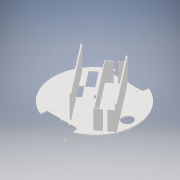
# Autodesk Inventor part: DonjaKonstrukcija_v.5.0
Saved by Autodesk Inventor 2020 (Build 240168000, 168)
## iProperties
Created: 2020-12-12
Part Number: DonjaKonstrukcija_v.5.0
Material: Generic
Document SubType Name: Modeling
Designer: Sičaja
Density: 1 g/cm^3
Appearance: Default
Author: Sičaja
Autodesk Inventor part; units mm, degrees
ref_plane "YZ Plane" through (0, 0, 0) normal (1, 0, 0) x (0, 1, 0)
ref_plane "XZ Plane" through (0, 0, 0) normal (0, 1, 0) x (-1, 0, 0)
ref_plane "XY Plane" through (0, 0, 0) normal (0, 0, 1) x (1, 0, 0)
sketch "Sketch1" plane through (0, 0, 0) normal (0, 1, 0) x (-1, 0, 0)
  arc A0 (125.0036, -29.4917) -> (126.5876, -26.2706) centre (125.0036, -27.4917) ccw projected
  line L0 (126.5876, -26.2706) -> (124.622, -23.7208) projected
  arc A1 (124.622, -23.7208) -> (122.2517, -23.1029) centre (123.038, -24.9419) ccw projected
  arc A2 (119.8815, -22.485) -> (122.2517, -23.1029) centre (121.4655, -21.264) ccw projected
  line L1 (119.8815, -22.485) -> (109.257, -8.7027) projected
  arc A3 (109.257, -8.7027) -> (107.673, -7.9237) centre (107.673, -9.9237) ccw projected
  line L2 (107.673, -7.9237) -> (105.1478, -7.9237) projected
  arc A4 (105.1478, -7.9237) -> (103.5638, -11.1448) centre (105.1478, -9.9237) ccw projected
  line L3 (103.5638, -11.1448) -> (117.1065, -28.7128) projected
  arc A5 (117.1065, -28.7128) -> (118.6904, -29.4917) centre (118.6904, -27.4917) ccw projected
  line L4 (118.6904, -29.4917) -> (125.0036, -29.4917) projected
  arc A6 (88.5004, 50.076) -> (88.5004, -87.4914) centre (118.3968, -18.7077) ccw projected
  line L5 (88.5004, 50.076) -> (90.9141, 40.0763) projected
  line L6 (90.9141, 40.0763) -> (103.8135, 40.0763) projected
  line L7 (103.8135, 40.0763) -> (103.8135, 42.0763) projected
  line L8 (103.8135, 42.0763) -> (105.8135, 42.0763) projected
  line L9 (105.8135, 42.0763) -> (105.8135, 40.0763) projected
  line L10 (105.8135, 40.0763) -> (117.3968, 40.0763) projected
  line L11 (117.3968, 40.0763) -> (117.3968, 42.0763) projected
  line L12 (117.3968, 42.0763) -> (119.3968, 42.0763) projected
  line L13 (119.3968, 42.0763) -> (119.3968, 40.0763) projected
  line L14 (119.3968, 40.0763) -> (145.8796, 40.0763) projected
  line L15 (145.8796, 40.0763) -> (148.2933, 50.076) projected
  arc A7 (148.2933, -87.4914) -> (148.2933, 50.076) centre (118.3968, -18.7077) ccw projected
  line L16 (148.2933, -87.4914) -> (145.8796, -77.4917) projected
  line L17 (145.8796, -77.4917) -> (119.3968, -77.4917) projected
  line L18 (119.3968, -77.4917) -> (119.3968, -79.4917) projected
  line L19 (119.3968, -79.4917) -> (117.3968, -79.4917) projected
  line L20 (117.3968, -79.4917) -> (117.3968, -77.4917) projected
  line L21 (117.3968, -77.4917) -> (90.9141, -77.4917) projected
  line L22 (90.9141, -77.4917) -> (88.5004, -87.4914) projected
  arc A8 (159.9383, -25.3226) -> (160.3012, -22.5175) centre (158.7173, -23.7386) ccw projected
  line L23 (160.3012, -22.5175) -> (147.6614, -6.1208) projected
  arc A9 (147.6614, -6.1208) -> (144.8563, -5.7578) centre (146.0774, -7.3418) ccw projected
  line L24 (144.8563, -5.7578) -> (136.9424, -11.8585) projected
  arc A10 (136.9424, -11.8585) -> (136.5795, -14.6635) centre (138.1635, -13.4424) ccw projected
  line L25 (136.5795, -14.6635) -> (149.2193, -31.0603) projected
  arc A11 (149.2193, -31.0603) -> (152.0244, -31.4232) centre (150.8033, -29.8392) ccw projected
  line L26 (152.0244, -31.4232) -> (159.9383, -25.3226) projected
  line L27 (160.2581, -68.311) -> (170.554, -60.3742) projected
  line L28 (170.554, -60.3742) -> (149.198, -32.6705) projected
  line L29 (149.198, -32.6705) -> (138.9021, -40.6074) projected
  line L30 (138.9021, -40.6074) -> (160.2581, -68.311) projected
  circle A12 centre (95.126, 34.6643) radius 1 projected
  circle A13 centre (141.6676, -72.0797) radius 1 projected
  circle A14 centre (141.6676, 34.6643) radius 1 projected
  circle A15 centre (95.126, -72.0797) radius 1 projected
  line L31 (108.9507, 33.0198) -> (177.0722, -55.3494) projected
  line L32 (177.0722, -55.3494) -> (178.6562, -54.1284) projected
  line L33 (178.6562, -54.1284) -> (110.5346, 34.2409) projected
  line L34 (110.5346, 34.2409) -> (108.9507, 33.0198) projected
  point P0 (0, 0)
extrude "DnoKonstrukcije" add sketch "Sketch1" along normal blind 2 contours L5 L6 L7 L8 L9 L10 L11 L12 L13 L14 L15 A7 L16 L17 L18 L19 L20 L21 L22 A6 | L33 L32 L31 L26 | L24 L31 L34 L33
sketch "Sketch6" plane through (0, 2, 0) normal (0, 1, 0) x (1, 0, 0)
  line L0 (-63.4991, -21.1731) -> (-64.1097, -20.3811) projected
  line L1 (-64.1097, -20.3811) -> (-72.8216, -27.0969) projected
  line L2 (-72.8216, -27.0969) -> (-137.5376, 56.8545) projected
  line L3 (-137.5376, 56.8545) -> (-128.6995, 63.6676) projected
  line L4 (-128.6995, 63.6676) -> (-129.31, 64.4595) projected
  line L5 (-129.31, 64.4595) -> (-138.9401, 57.036) projected
  line L6 (-73.0031, -28.4994) -> (-138.9401, 57.036) projected
  line L7 (-63.4991, -21.1731) -> (-73.0031, -28.4994) projected
  line L8 (-50.8272, -11.4047) -> (-51.4378, -10.6127) projected
  line L9 (-51.4378, -10.6127) -> (-59.3577, -16.7179) projected
  line L10 (-59.3577, -16.7179) -> (-58.7472, -17.5099) projected
  line L11 (-50.8272, -11.4047) -> (-58.7472, -17.5099) projected
  line L12 (-115.1802, 75.3518) -> (-116.7642, 74.1308) projected
  line L13 (-116.7642, 74.1308) -> (-50.8272, -11.4047) projected
  line L14 (-50.8272, -11.4047) -> (-49.2432, -10.1836) projected
  line L15 (-49.2432, -10.1836) -> (-115.1802, 75.3518) projected
  line L16 (-116.1537, 73.3388) -> (-116.7642, 74.1308) projected
  line L17 (-116.7642, 74.1308) -> (-124.6842, 68.0255) projected
  line L18 (-124.6842, 68.0255) -> (-124.0737, 67.2335) projected
  line L19 (-124.0737, 67.2335) -> (-116.1537, 73.3388) projected
  point P0 (0, 0)
extrude "DrzacZaBateriju" add sketch "Sketch6" along normal blind 34
sketch "Sketch7" plane through (0, 36, 0) normal (0, 1, 0) x (1, 0, 0)
  line L0 (-49.2432, -10.1836) -> (-115.1802, 75.3518) projected
  line L1 (-115.1802, 75.3518) -> (-124.6842, 68.0255) projected
  line L2 (-124.6842, 68.0255) -> (-124.0737, 67.2335) projected
  line L3 (-124.0737, 67.2335) -> (-116.1537, 73.3388) projected
  line L4 (-116.1537, 73.3388) -> (-51.4378, -10.6127) projected
  line L5 (-51.4378, -10.6127) -> (-59.3577, -16.7179) projected
  line L6 (-59.3577, -16.7179) -> (-58.7472, -17.5099) projected
  line L7 (-58.7472, -17.5099) -> (-49.2432, -10.1836) projected
  line L8 (-124.0737, 67.2335) -> (-116.1537, 73.3388) projected
  line L9 (-116.1537, 73.3388) -> (-116.7642, 74.1308)
  line L10 (-51.4378, -10.6127) -> (-59.3577, -16.7179) projected
  line L11 (-51.4378, -10.6127) -> (-50.8272, -11.4047)
  line L12 (-58.7472, -17.5099) -> (-49.2432, -10.1836) projected
  point P0 (0, 0)
  constraints: 4 end point, 3 point on line, 1 perpendicular
extrude "DrzacZaTeensy" add sketch "Sketch7" along normal blind 10 contours L7 L11 L4 L9 L1 L0
sketch "Sketch8" plane through (0, 2, 0) normal (0, 1, 0) x (1, 0, 0)
  line L0 (-108.9507, -33.0198) -> (-177.0722, 55.3494) projected
  line L1 (-177.0722, 55.3494) -> (-178.6562, 54.1284) projected
  line L2 (-178.6562, 54.1284) -> (-110.5346, -34.2409) projected
  line L3 (-110.5346, -34.2409) -> (-108.9507, -33.0198) projected
  point P0 (0, 0)
extrude "DrzacZaPDB" add sketch "Sketch8" along normal blind 42
sketch "Sketch10" plane through (-110.5346, 2, 34.2409) normal (-0.7919947, 0, 0.6105279) x (0.6105279, 0, 0.7919947)
  point P0 (40.3659, -2)
sketch "Sketch11" plane through (-110.5346, 2, 34.2409) normal (-0.7919947, 0, 0.6105279) x (0.6105279, 0, 0.7919947)
  circle A0 centre (-42.3, 37.7) radius 1 projected
  circle A1 centre (-2.3, 37.7) radius 1 projected
  circle A2 centre (-42.3, 7.7) radius 1 projected
  point P0 (40.3659, -2)
extrude "RupeZaPDBSEkranom" cut sketch "Sketch11" against normal blind 2
sketch "Sketch12" plane through (-110.5346, 2, 34.2409) normal (-0.7919947, 0, 0.6105279) x (0.6105279, 0, 0.7919947)
  line L0 (-45.4471, 40.0341) -> (-75.4471, 40.0341)
  line L1 (-75.4471, 40.0341) -> (-75.4471, 5.0341)
  line L2 (-75.4471, 5.0341) -> (-45.4471, 5.0341)
  line L3 (-45.4471, 5.0341) -> (-45.4471, 40.0341)
  line L4 (-71.9471, 37.5341) -> (-48.9471, 37.5341)
  line L5 (-47.9471, 36.5341) -> (-47.9471, 8.5341)
  line L6 (-48.9471, 7.5341) -> (-71.9471, 7.5341)
  line L7 (-72.9471, 8.5341) -> (-72.9471, 36.5341)
  circle A0 centre (-72.9471, 37.5341) radius 1
  circle A1 centre (-47.9471, 37.5341) radius 1
  circle A2 centre (-72.9471, 7.5341) radius 1
  circle A3 centre (-47.9471, 7.5341) radius 1
  point P0 (40.3659, -2)
  dimension "d16" = 30
  dimension "d17" = 35
  dimension "d18" = 2.5
  dimension "d19" = 2
  dimension "d20" = 2
  dimension "d21" = 2
  dimension "d22" = 2
  constraints: 16 end point, 8 point on circle, 4 centre point, 4 parallel, 2 perpendicular, 1 horizontal
  measures "d16" distance of L2.end L1.end
  measures "d17" distance of L1.end L0.end
  measures "d18" distance between parallel lines of L0 L4
  measures "d19" diameter of A0
  measures "d20" diameter of A1
  measures "d21" diameter of A2
  measures "d22" diameter of A3
extrude "RupeZaDriverMotora" cut sketch "Sketch12" against normal blind 2 contours A0 | A1 | A2 | A3
sketch "Sketch15" plane through (-110.5346, 2, 34.2409) normal (-0.7919947, 0, 0.6105279) x (0.6105279, 0, 0.7919947)
  line L0 (-110.3095, 40.1713) -> (-80.3095, 40.1713)
  line L1 (-80.3095, 40.1713) -> (-80.3095, 5.1713)
  line L2 (-80.3095, 5.1713) -> (-110.3095, 5.1713)
  line L3 (-110.3095, 5.1713) -> (-110.3095, 40.1713)
  line L4 (-83.8095, 37.6713) -> (-106.8095, 37.6713)
  line L5 (-107.8095, 36.6713) -> (-107.8095, 8.6713)
  line L6 (-106.8095, 7.6713) -> (-83.8095, 7.6713)
  line L7 (-82.8095, 8.6713) -> (-82.8095, 36.6713)
  circle A0 centre (-107.8095, 37.6713) radius 1
  circle A1 centre (-82.8095, 37.6713) radius 1
  circle A2 centre (-107.8095, 7.6713) radius 1
  circle A3 centre (-82.8095, 7.6713) radius 1
  point P0 (40.3659, -2)
  dimension "d25" = 30
  dimension "d26" = 35
  dimension "d27" = 2.5
  dimension "d28" = 2
  dimension "d29" = 2
  dimension "d30" = 2
  dimension "d31" = 2
  constraints: 16 end point, 8 point on circle, 4 centre point, 4 parallel, 2 perpendicular, 1 horizontal
  measures "d25" distance of L1.end L2.end
  measures "d26" distance of L0.end L1.end
  measures "d27" distance between parallel lines of L0 L4
  measures "d28" diameter of A0
  measures "d29" diameter of A1
  measures "d30" diameter of A2
  measures "d31" diameter of A3
extrude "RupeZaPDB" cut sketch "Sketch15" against normal blind 2 contours A1 | A0 | A3 | A2
sketch "Sketch16" plane through (-115.1802, 2, -75.3518) normal (0.7919947, 0, -0.6105279) x (-0.6105279, 0, -0.7919947)
  line L0 (-89.0986, 42.7042) -> (-24.0986, 42.7042)
  line L1 (-24.0986, 42.7042) -> (-24.0986, 7.7042)
  line L2 (-24.0986, 7.7042) -> (-89.0986, 7.7042)
  line L3 (-89.0986, 7.7042) -> (-89.0986, 42.7042)
  line L4 (-85.5986, 10.2042) -> (-27.5986, 10.2042)
  line L5 (-26.5986, 11.2042) -> (-26.5986, 39.2042)
  line L6 (-27.5986, 40.2042) -> (-85.5986, 40.2042)
  line L7 (-86.5986, 39.2042) -> (-86.5986, 11.2042)
  circle A0 centre (-86.5986, 40.2042) radius 1
  circle A1 centre (-26.5986, 40.2042) radius 1
  circle A2 centre (-86.5986, 10.2042) radius 1
  circle A3 centre (-26.5986, 10.2042) radius 1
  point P0 (-129.999, -2)
  dimension "d34" = 65
  dimension "d35" = 35
  dimension "d36" = 2.5
  dimension "d37" = 2
  dimension "d38" = 2
  dimension "d39" = 2
  dimension "d40" = 2
  constraints: 16 end point, 8 point on circle, 4 centre point, 4 parallel, 2 perpendicular, 1 horizontal
  measures "d34" distance of L1.end L2.end
  measures "d35" distance of L0.end L1.end
  measures "d36" distance between parallel lines of L2 L4
  measures "d37" diameter of A0
  measures "d38" diameter of A1
  measures "d39" diameter of A2
  measures "d40" diameter of A3
extrude "RupeZaTeensy" cut sketch "Sketch16" against normal blind 2 contours A2 | A3 | A0 | A1
sketch "Sketch17" plane through (0, 0, 0) normal (0, -1, 0) x (1, 0, 0)
  line L0 (-90.9141, 40.0763) -> (-88.5004, 50.076) projected
  line L1 (-88.5004, -87.4914) -> (-90.9141, -77.4917) projected
  line L2 (-90.9141, 40.0763) -> (-90.9141, -77.4917)
  line L3 (-90.9141, 40.0763) -> (-90.9141, -18.7077)
  line L4 (-90.9141, -18.7077) -> (-43.3968, -18.7077)
  arc A0 (-88.5004, -87.4914) -> (-88.5004, 50.076) centre (-118.3968, -18.7077) ccw projected
  circle A1 centre (-62.2603, -18.7077) radius 9.5
  point P0 (0, 0)
  dimension "d43" = 58.784
  dimension "d44" = 19
  constraints: 6 end point, 1 centre point, 1 midpoint, 1 perpendicular, 1 point on circle, 1 vertical
  measures "d43" distance of L0.start L3.end
  measures "d44" diameter of A1
extrude "RupaZaLezaj" cut sketch "Sketch17" against normal blind 2 contours A1 L4 | L4 A1
body "Solid1"
